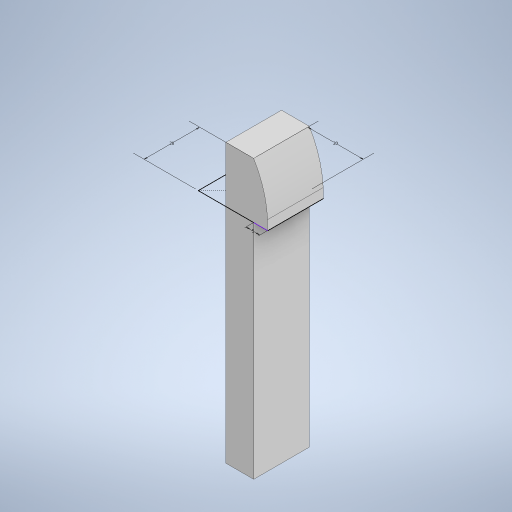
# Autodesk Inventor part: 찐탄두조절자
Saved by Autodesk Inventor 2023 (Build 270158000, 158)
## iProperties
Created: 2023-10-30
Part Number: 찐탄두조절자
Material: 일반
Document SubType Name: Modeling
Designer: rlatk
Density: 1 g/cm^3
Appearance: 기본값
Author: rlatk
Autodesk Inventor part; units mm, degrees
ref_plane "YZ Plane" through (0, 0, 0) normal (1, 0, 0) x (0, 1, 0)
ref_plane "XZ Plane" through (0, 0, 0) normal (0, 1, 0) x (-1, 0, 0)
ref_plane "XY Plane" through (0, 0, 0) normal (0, 0, 1) x (1, 0, 0)
sketch "스케치1" plane through (0, 0, 0) normal (0, 1, 0) x (-1, 0, 0)
  line L0 (-10, 10) -> (10, 10)
  line L1 (10, 10) -> (10, -10)
  line L2 (10, -10) -> (-10, -10)
  line L3 (-10, -10) -> (-10, 10)
  line L4 (-10, 10) -> (10, -10) construction
  line L5 (10, 10) -> (-10, -10) construction
  line L6 (-10, -10) -> (-15, -10)
  line L7 (-15, -10) -> (-15, 10)
  line L8 (-15, 10) -> (-10, 10)
  line L9 (-10, 10) -> (-10, -10)
  point P0 (0, 0)
  dimension "d0" = 20
  dimension "d1" = 20
  dimension "d2" = 5
  constraints: 20 end point, 4 parallel, 2 horizontal, 2 midpoint, 2 perpendicular
  measures "d0" distance of L1.end L2.end
  measures "d1" distance of L0.end L1.end
  measures "d2" distance of L7.end L8.end
extrude "돌출1" add sketch "스케치1" along normal blind 20
extrude "돌출2" add sketch "스케치1" against normal blind 80 contours L0 L1 L2 L3
sketch "스케치2" plane through (-10, 20, -10) normal (-1, 0, 0) x (0, 0, 1)
  line L0 (20, -100) -> (20, 0) projected
  line L1 (0, 0) -> (20, 0) projected
  line L2 (0, 0) -> (0, -100) projected
  line L3 (20, -100) -> (0, -100) projected
  circle A0 centre (10, -91) radius 4.5
  point P0 (10, -20)
  dimension "d7" = 9
  dimension "d8" = 9
  constraints: 1 centre point
  measures "d7" diameter of A0
  measures "d8" distance from line of L3 A0.centre
sketch "스케치3" plane through (-10, 20, 10) normal (0, 0, 1) x (1, 0, 0)
  line L0 (20, -20) -> (25, -20) projected
  line L1 (25, -20) -> (25, 0) projected
  line L2 (0, 0) -> (25, 0) projected
  line L3 (0, -100) -> (0, 0) projected
  line L4 (20, -100) -> (0, -100) projected
  line L5 (20, -20) -> (20, -100) projected
  line L6 (25, -20) -> (25, 0) projected
  line L7 (25, 0) -> (0, 0) projected
  arc A0 (25, -20) -> (20, 0) centre (-10.6945, -18.2986) ccw
  line L8 (20, 0) -> (25, 0)
  line L9 (25, 0) -> (25, -20)
  point P0 (10, -20)
  point P1 (20, 0)
  point P2 (25, -16.5972)
  constraints: 4 end point, 2 collinear, 2 point on circle, 1 centre point, 1 point on line
extrude "돌출4" cut sketch "스케치3" against normal blind 20 contours A0 L2 L1
extrude "돌출5" cut sketch "스케치2" against normal blind 10
sketch "스케치4" plane through (-10, -71, 0) normal (-1, 0, 0) x (0, 0, 1)
  circle A0 centre (0, 0) radius 4.5 projected
  point P0 (0, 71)
extrude "돌출6" cut sketch "스케치4" against normal blind 15
